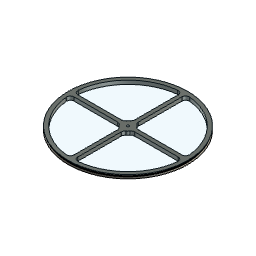
wheel v6 (Autodesk Fusion 360 design; units mm, degrees)
Autodesk Fusion 360 part; units mm, degrees
sketch "Sketch1" plane through (0, 0, 0) normal (0, 0, 1) x (1, 0, 0)
  circle A0 centre (0, 0) radius 41.275
  circle A1 centre (0, 0) radius 38.735
  circle A2 centre (0, 0) radius 4.445
  dimension "d1" = 82.55
  dimension "d2" = 77.47
  dimension "d5" = 8.89
  constraint coincident A0.centre A1.centre
  measures "d1" diameter of A0
  measures "d2" diameter of A1
  measures "d5" diameter of A2
extrude "Extrude1" add sketch "Sketch1" along normal blind 2.54 makes body 1 at (41.2237, -2.0574, 1.6933) makes body 2 at (4.4229, -0.4426, 0.8467)
sketch "Sketch4" plane through (0, 0, 0) normal (0, 0, 1) x (1, 0, 0)
  line L0 (-1.27, 39.37) -> (1.27, 39.37)
  line L1 (1.27, 39.37) -> (1.27, 1.27)
  line L2 (1.27, 1.27) -> (-1.27, 1.27)
  line L3 (-1.27, 1.27) -> (-1.27, 39.37)
  dimension "d12" = 2.54
  dimension "d13" = 1.27
  dimension "d14" = 38.1
  dimension "d15" = 1.27
  constraint horizontal L0
  constraint vertical L1
  constraint horizontal L2
  constraint vertical L3
  measures "d12" distance of L1.end L2.end
  measures "d13" horizontal distance of origin L1.end
  measures "d14" distance of L0.end L1.end
  measures "d15" vertical distance of origin L2.end
extrude "Extrude3" add sketch "Sketch4" along normal blind 2.54 separate body makes body 3
pattern_circular "C-Pattern1" count 4 over 360 about axis through (0, 0, 1.75) along (0, 0, 1) of bodies 3 makes body 4 at (-26.67, 1.27, 0.8467) makes body 5 at (-1.27, -26.67, 0.8467) makes body 6 at (26.67, -1.27, 0.8467)
combine "Combine1" operation add target body 3 tool bodies 1 2 6 5 4
fillet "Fillet1" radius 2.54 8 edges at (4.2597, 1.27, 1.27) (1.27, 4.2597, 1.27) (-1.27, 4.2597, 1.27) (-4.2597, 1.27, 1.27) (-4.2597, -1.27, 1.27) (-1.27, -4.2597, 1.27) (1.27, -4.2597, 1.27) (4.2597, -1.27, 1.27) on bodies 3
fillet "Fillet2" radius 2.54 8 edges at (1.27, -38.7142, 1.27) (-1.27, -38.7142, 1.27) (-38.7142, -1.27, 1.27) (-38.7142, 1.27, 1.27) (-1.27, 38.7142, 1.27) (1.27, 38.7142, 1.27) (38.7142, 1.27, 1.27) (38.7142, -1.27, 1.27) on bodies 3
sketch "Sketch5" plane through (0, 0, 0) normal (1, 0, 0) x (0, 1, 0)
  line L0 (-41.275, 2.54) -> (-40.8209, 2.159)
  line L1 (-40.8209, 2.159) -> (-40.8209, 0.381)
  line L2 (-40.8209, 0.381) -> (-41.275, 0)
  line L3 (-41.275, 2.54) -> (-41.275, 0)
  dimension "d24" = 1.778
  dimension "d25" = 2.54
  dimension "d26" = 130
  dimension "d27" = 130
  dimension "d28" = 41.275
  constraint vertical L1
  constraint vertical L3
  constraint horizontal origin L2.end
  measures "d24" distance of L0.end L1.end
  measures "d25" distance of L0.start L2.end
  measures "d26" angle of L0 L1
  measures "d27" angle of L1 L2
  measures "d28" horizontal distance of origin L2.end
revolve "Revolve1" cut sketch "Sketch5" angle 360 about axis through (0, 0, 1.75) along (0, 0, 1) bodies 3
hole "Hole1" at (0, 0, 2.54) direction (0, 0, -1) diameter 1.6256 depth 6.35 tip angle 118 bodies 3
thread "Thread1" "ISO Metric profile 2.0 M2x0.4 6H" thread offset 0 thread depth 5.9436
sketch "Sketch6" plane through (0, 0, 2.54) normal (0, 0, 1) x (-1, 0, 0)
  circle A0 centre (0, 0) radius 0.8115
  arc A1 (4.0774, -38.5198) -> (38.5198, -4.0774) centre (0, 0) ccw
  arc A2 (1.27, -35.9939) -> (4.0774, -38.5198) centre (3.81, -35.9939) ccw
  line L0 (1.27, -35.9939) -> (1.27, -5.8544)
  arc A3 (2.4245, -3.7255) -> (1.27, -5.8544) centre (3.81, -5.8544) ccw
  arc A4 (2.4245, -3.7255) -> (3.7255, -2.4245) centre (0, 0) ccw
  arc A5 (5.8544, -1.27) -> (3.7255, -2.4245) centre (5.8544, -3.81) ccw
  line L1 (5.8544, -1.27) -> (35.9939, -1.27)
  arc A6 (38.5198, -4.0774) -> (35.9939, -1.27) centre (35.9939, -3.81) ccw
  line L2 (-35.9939, -1.27) -> (-5.8544, -1.27)
  arc A7 (-3.7255, -2.4245) -> (-5.8544, -1.27) centre (-5.8544, -3.81) ccw
  arc A8 (-3.7255, -2.4245) -> (-2.4245, -3.7255) centre (0, 0) ccw
  arc A9 (-1.27, -5.8544) -> (-2.4245, -3.7255) centre (-3.81, -5.8544) ccw
  line L3 (-1.27, -5.8544) -> (-1.27, -35.9939)
  arc A10 (-4.0774, -38.5198) -> (-1.27, -35.9939) centre (-3.81, -35.9939) ccw
  arc A11 (-38.5198, -4.0774) -> (-4.0774, -38.5198) centre (0, 0) ccw
  arc A12 (-35.9939, -1.27) -> (-38.5198, -4.0774) centre (-35.9939, -3.81) ccw
  circle A13 centre (0, 0) radius 41.275
  line L4 (-1.27, 35.9939) -> (-1.27, 5.8544)
  arc A14 (-2.4245, 3.7255) -> (-1.27, 5.8544) centre (-3.81, 5.8544) ccw
  arc A15 (-2.4245, 3.7255) -> (-3.7255, 2.4245) centre (0, 0) ccw
  arc A16 (-5.8544, 1.27) -> (-3.7255, 2.4245) centre (-5.8544, 3.81) ccw
  line L5 (-5.8544, 1.27) -> (-35.9939, 1.27)
  arc A17 (-38.5198, 4.0774) -> (-35.9939, 1.27) centre (-35.9939, 3.81) ccw
  arc A18 (-4.0774, 38.5198) -> (-38.5198, 4.0774) centre (0, 0) ccw
  arc A19 (-1.27, 35.9939) -> (-4.0774, 38.5198) centre (-3.81, 35.9939) ccw
  line L6 (35.9939, 1.27) -> (5.8544, 1.27)
  arc A20 (3.7255, 2.4245) -> (5.8544, 1.27) centre (5.8544, 3.81) ccw
  arc A21 (3.7255, 2.4245) -> (2.4245, 3.7255) centre (0, 0) ccw
  arc A22 (1.27, 5.8544) -> (2.4245, 3.7255) centre (3.81, 5.8544) ccw
  line L7 (1.27, 5.8544) -> (1.27, 35.9939)
  arc A23 (4.0774, 38.5198) -> (1.27, 35.9939) centre (3.81, 35.9939) ccw
  arc A24 (38.5198, 4.0774) -> (4.0774, 38.5198) centre (0, 0) ccw
  arc A25 (35.9939, 1.27) -> (38.5198, 4.0774) centre (35.9939, 3.81) ccw
fillet "Fillet3" radius 1.27 2 edges at (-38.0585, -14.7615, 2.159) (-38.0585, -14.7615, 0.381) on bodies 3
sketch "Sketch8" plane through (0, 0, 0) normal (0, 0, -1) x (1, 0, 0)
  circle A0 centre (0, 0) radius 0.8115
  arc A1 (-1.27, 35.9939) -> (-4.0774, 38.5198) centre (-3.81, 35.9939) ccw
  line L0 (-1.27, 35.9939) -> (-1.27, 5.8544)
  arc A2 (-2.4245, 3.7255) -> (-1.27, 5.8544) centre (-3.81, 5.8544) ccw
  arc A3 (-2.4245, 3.7255) -> (-3.7255, 2.4245) centre (0, 0) ccw
  arc A4 (-5.8544, 1.27) -> (-3.7255, 2.4245) centre (-5.8544, 3.81) ccw
  line L1 (-5.8544, 1.27) -> (-35.9939, 1.27)
  arc A5 (-38.5198, 4.0774) -> (-35.9939, 1.27) centre (-35.9939, 3.81) ccw
  arc A6 (-4.0774, 38.5198) -> (-38.5198, 4.0774) centre (0, 0) ccw
  line L2 (-35.9939, -1.27) -> (-5.8544, -1.27)
  arc A7 (-3.7255, -2.4245) -> (-5.8544, -1.27) centre (-5.8544, -3.81) ccw
  arc A8 (-3.7255, -2.4245) -> (-2.4245, -3.7255) centre (0, 0) ccw
  arc A9 (-1.27, -5.8544) -> (-2.4245, -3.7255) centre (-3.81, -5.8544) ccw
  line L3 (-1.27, -5.8544) -> (-1.27, -35.9939)
  arc A10 (-4.0774, -38.5198) -> (-1.27, -35.9939) centre (-3.81, -35.9939) ccw
  arc A11 (-38.5198, -4.0774) -> (-4.0774, -38.5198) centre (0, 0) ccw
  arc A12 (-35.9939, -1.27) -> (-38.5198, -4.0774) centre (-35.9939, -3.81) ccw
  arc A13 (35.9939, 1.27) -> (38.5198, 4.0774) centre (35.9939, 3.81) ccw
  line L4 (35.9939, 1.27) -> (5.8544, 1.27)
  arc A14 (3.7255, 2.4245) -> (5.8544, 1.27) centre (5.8544, 3.81) ccw
  arc A15 (3.7255, 2.4245) -> (2.4245, 3.7255) centre (0, 0) ccw
  arc A16 (1.27, 5.8544) -> (2.4245, 3.7255) centre (3.81, 5.8544) ccw
  line L5 (1.27, 5.8544) -> (1.27, 35.9939)
  arc A17 (4.0774, 38.5198) -> (1.27, 35.9939) centre (3.81, 35.9939) ccw
  arc A18 (38.5198, 4.0774) -> (4.0774, 38.5198) centre (0, 0) ccw
  line L6 (1.27, -35.9939) -> (1.27, -5.8544)
  arc A19 (2.4245, -3.7255) -> (1.27, -5.8544) centre (3.81, -5.8544) ccw
  arc A20 (2.4245, -3.7255) -> (3.7255, -2.4245) centre (0, 0) ccw
  arc A21 (5.8544, -1.27) -> (3.7255, -2.4245) centre (5.8544, -3.81) ccw
  line L7 (5.8544, -1.27) -> (35.9939, -1.27)
  arc A22 (38.5198, -4.0774) -> (35.9939, -1.27) centre (35.9939, -3.81) ccw
  arc A23 (4.0774, -38.5198) -> (38.5198, -4.0774) centre (0, 0) ccw
  arc A24 (1.27, -35.9939) -> (4.0774, -38.5198) centre (3.81, -35.9939) ccw
  circle A25 centre (0, 0) radius 41.275
  line L8 (-2.0319, 1.778) -> (2.0319, 1.778)
  line L9 (-2.0319, -1.778) -> (2.0319, -1.778)
  arc A26 (-2.0319, 1.778) -> (-2.0319, -1.778) centre (0, 0) ccw
  arc A27 (2.0319, -1.778) -> (2.0319, 1.778) centre (0, 0) ccw
  dimension "d42" = 5.4
  dimension "d43" = 3.556
  constraint concentric A0 A26
  constraint horizontal L8
  constraint coincident L9.end A26
  constraint horizontal L9
  constraint vertical L8.start L9.start
  constraint concentric A26 A27
  measures "d42" diameter of A26
  measures "d43" distance of L8 L9
extrude "Extrude4" cut sketch "Sketch8" against normal blind 1.27 contours L8 L9 A26 A27 bodies 3
